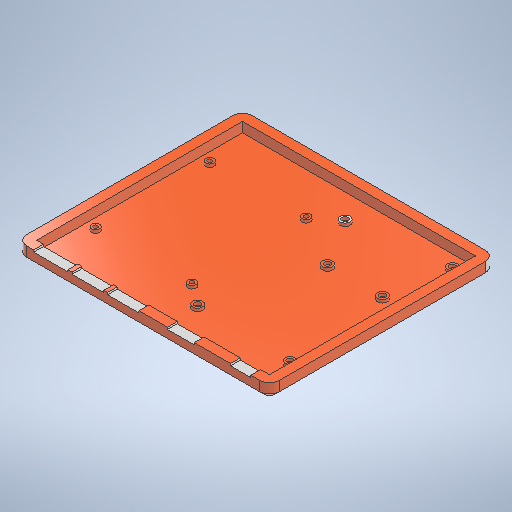
# Autodesk Inventor part: Electronic Base - Layered
Saved by Autodesk Inventor 2025.2 (Build 292293000, 293)
## iProperties
Created: 2025-02-05
Part Number: Electronic Base - Layered
Material: Generic
Document SubType Name: Modeling
Designer: caomi
Density: 1 g/cm^3
Appearance: Default
Author: caomi
Autodesk Inventor part; units mm, degrees
ref_plane "YZ Plane" through (0, 0, 0) normal (1, 0, 0) x (0, 1, 0)
ref_plane "XZ Plane" through (0, 0, 0) normal (0, 1, 0) x (-1, 0, 0)
ref_plane "XY Plane" through (0, 0, 0) normal (0, 0, 1) x (1, 0, 0)
sketch "Sketch1" plane through (0, 0, 0) normal (0, 1, 0) x (-1, 0, 0)
  line L0 (128.34, 114.6) -> (0, 114.6)
  line L1 (0, 114.6) -> (0, 0)
  line L2 (0, 0) -> (128.34, 0)
  line L3 (128.34, 0) -> (128.34, 114.6)
  line L4 (121.34, 23.6) -> (65.34, 23.6) construction
  line L5 (65.34, 23.6) -> (65.34, 108.6) construction
  line L6 (65.34, 108.6) -> (121.34, 108.6) construction
  line L7 (121.34, 108.6) -> (121.34, 23.6) construction
  circle A0 centre (117.84, 27.1) radius 1.1
  circle A1 centre (117.84, 85.1) radius 1.1
  circle A2 centre (68.84, 27.1) radius 1.1
  circle A3 centre (68.84, 85.1) radius 1.1
  line L8 (0, 0) -> (-136.9444, 0) construction
  line L9 (0, 0) -> (0, -49.9102) construction
  circle A4 centre (117.84, 27.1) radius 2.1
  circle A5 centre (117.84, 85.1) radius 2.1
  circle A6 centre (68.84, 27.1) radius 2.1
  circle A7 centre (68.84, 85.1) radius 2.1
  line L10 (123.34, 5) -> (5, 5)
  line L11 (5, 5) -> (5, 109.6)
  line L12 (5, 109.6) -> (123.34, 109.6)
  line L13 (123.34, 109.6) -> (123.34, 5)
  line L14 (60.34, 7) -> (7, 7) construction
  line L15 (7, 7) -> (7, 108.6) construction
  line L16 (7, 108.6) -> (60.34, 108.6) construction
  line L17 (60.34, 108.6) -> (60.34, 7) construction
  circle A8 centre (57.8, 18.43) radius 2.55
  circle A9 centre (57.8, 18.43) radius 1.55
  circle A10 centre (42.56, 42.56) radius 2.55
  circle A11 centre (42.56, 42.56) radius 1.55
  circle A12 centre (57.8, 93.36) radius 1.55
  circle A13 centre (14.62, 42.56) radius 2.55
  circle A14 centre (57.8, 93.36) radius 2.55
  circle A15 centre (14.62, 42.56) radius 1.55
  circle A16 centre (9.54, 12.08) radius 2.55
  circle A17 centre (9.54, 12.08) radius 1.55
  circle A18 centre (9.54, 94.63) radius 2.55
  circle A19 centre (9.54, 94.63) radius 1.55
  point P0 (121.34, 66.1)
  point P1 (7, 57.8)
  point P2 (1.5544, 63)
  point P3 (2.0056, 63)
  point P4 (82.8344, 63)
  point P5 (83.2856, 63)
  point P6 (33.67, 108.6)
  dimension "d10" = 2.2
  dimension "d48" = 101.6
  dimension "d49" = 53.34
  dimension "d59" = 5
  dimension "d62" = 3.1
  dimension "d63" = 1
  dimension "d73" = 5
  dimension "d79" = 5
  dimension "d81" = 2
  dimension "d82" = 2.54
  dimension "d83" = 15.24
  dimension "d84" = 90.17
  dimension "d85" = 96.52
  dimension "d86" = 50.8
  dimension "d87" = 66.04
  dimension "d88" = 17.78
  dimension "d89" = 45.72
  dimension "d90" = 13.97
  dimension "d91" = 85
  dimension "d92" = 58
  dimension "d95" = 1
  dimension "d96" = 3.5
  dimension "d97" = 3.5
  dimension "d98" = 3.5
  dimension "d99" = 56
  dimension "d100" = 2
  dimension "d101" = 2
  dimension "d102" = 5
  dimension "d103" = 5
  dimension "d120" = 1
  constraints: 36 end point, 20 centre point, 16 equal radius, 8 parallel, 6 coincident, 5 horizontal, 4 perpendicular, 4 vertical alignment, 3 horizontal alignment, 3 midpoint, 1 collinear, 1 vertical
  measures "d10" diameter of A0
  measures "d48" distance of L16.end L14.start
  measures "d49" distance of L15.end L16.end
  measures "d59" distance between parallel lines of L13 L3
  measures "d62" diameter of A9
  measures "d63" radial gap between concentric circles of A8 A9
  measures "d73" distance between parallel lines of L0 L12
  measures "d79" distance between parallel lines of L2 L10
  measures "d81" distance between parallel lines of L10 L14
  measures "d82" distance from line of L17 A12.centre
  measures "d83" distance from line of L16 A12.centre
  measures "d84" distance from line of L16 A9.centre
  measures "d85" distance from line of L16 A16.centre
  measures "d86" distance from line of L17 A17.centre
  measures "d87" distance from line of L16 A10.centre
  measures "d88" distance from line of L17 A10.centre
  measures "d89" distance from line of L17 A15.centre
  measures "d90" distance from line of L16 A18.centre
  measures "d91" distance of L4.end L5.end
  measures "d92" distance of A3.centre A2.centre
  measures "d95" radial gap between concentric circles of A4 A0
  measures "d96" distance from line of L4 A2.centre
  measures "d97" distance from line of L7 A0.centre
  measures "d98" distance from line of L5 A2.centre
  measures "d99" distance between parallel lines of L7 L5
  measures "d100" distance between parallel lines of L11 L15
  measures "d101" distance between parallel lines of L13 L7
  measures "d102" distance between parallel lines of L1 L11
  measures "d103" distance between parallel lines of L17 L5
  measures "d120" distance from line of L12 point (33.67, 108.6)
extrude "Extrusion1" add sketch "Sketch1" against normal blind 2 contours L3 L2 L1 L0 | A0 | A1 | A2 | A3 | A4 | A5 | A6 | A7 | L10 L11 L12 L13 | A8 | A9 | A10 | A11 | A12 | A13 | A14 | A15 | A16 | A17 | A18 | A19
extrude "Extrusion2" add sketch "Sketch1" along normal blind 5 contours L3 L2 L1 L0
extrude "Extrusion3" add sketch "Sketch1" along normal blind 1.5 contours A4 | A5 | A6 | A7 | A8 | A10 | A13 | A14 | A16 | A18
fillet "Fillet1" radius 5 4 edges at (-128.34, 1.5, 0) (0, 1.5, 114.6) (-128.34, 1.5, 114.6) (0, 1.5, 0)
chamfer "Chamfer1" distance 2 angle 45 7 edges at (-64.17, -2, 114.6) (-126.8755, -2, 113.1355) (-128.34, -2, 57.3) (-126.8755, -2, 1.4645) (-64.17, -2, 0) (0, -2, 57.3) (-1.4645, -2, 113.1355)
sketch "Sketch2" plane through (0, 5, 0) normal (0, 1, 0) x (1, 0, 0)
  line L0 (-123.34, -114.6) -> (-5, -114.6) projected
  line L1 (-5, -109.6) -> (-123.34, -109.6) projected
  line L2 (-119.84, -109.6) -> (-102.44, -109.6)
  line L3 (-102.44, -109.6) -> (-102.44, -114.6)
  line L4 (-102.44, -114.6) -> (-119.84, -114.6)
  line L5 (-119.84, -114.6) -> (-119.84, -109.6)
  line L6 (-100.34, -109.6) -> (-84.24, -109.6)
  line L7 (-84.24, -109.6) -> (-84.24, -114.6)
  line L8 (-84.24, -114.6) -> (-100.34, -114.6)
  line L9 (-100.34, -114.6) -> (-100.34, -109.6)
  line L10 (-82.34, -109.6) -> (-66.34, -109.6)
  line L11 (-66.34, -109.6) -> (-66.34, -114.6)
  line L12 (-66.34, -114.6) -> (-82.34, -114.6)
  line L13 (-82.34, -114.6) -> (-82.34, -109.6)
  line L14 (-51.84, -109.6) -> (-38.2, -109.6)
  line L15 (-38.2, -109.6) -> (-38.2, -114.6)
  line L16 (-38.2, -114.6) -> (-51.84, -114.6)
  line L17 (-51.84, -114.6) -> (-51.84, -109.6)
  line L18 (-121.34, -108.6) -> (-121.34, -23.6) construction
  line L19 (-60.34, -108.6) -> (-60.34, -7) construction
  line L20 (-19.84, -109.6) -> (-9.51, -109.6)
  line L21 (-9.51, -109.6) -> (-9.51, -114.6)
  line L22 (-9.51, -114.6) -> (-19.84, -114.6)
  line L23 (-19.84, -114.6) -> (-19.84, -109.6)
  point P0 (0, 0)
  point P1 (-9.51, -112.1)
  point P2 (-19.84, -114.6)
  point P3 (-51.84, -114.6)
  dimension "d104" = 17.4
  dimension "d107" = 16.1
  dimension "d109" = 16
  dimension "d113" = 13.64
  dimension "d114" = 1.5
  dimension "d115" = 21
  dimension "d116" = 39
  dimension "d117" = 8.5
  dimension "d118" = 40.5
  dimension "d119" = 10.33
  constraints: 40 end point, 10 parallel, 10 point on line, 5 horizontal, 5 perpendicular, 1 midpoint
  measures "d104" distance of L3.end L4.end
  measures "d107" distance of L7.end L8.end
  measures "d109" distance between parallel lines of L11 L13
  measures "d113" distance between parallel lines of L15 L17
  measures "d114" distance between parallel lines of L18 L5
  measures "d115" distance between parallel lines of L18 L9
  measures "d116" distance between parallel lines of L18 L13
  measures "d117" distance between parallel lines of L19 L17
  measures "d118" distance between parallel lines of L19 L23
  measures "d119" distance from line of point (-9.51, -112.1) L23
extrude "Extrusion4" cut sketch "Sketch2" against normal blind 1 contours L5 L1 L3 L0 | L9 L1 L7 L0 | L13 L1 L11 L0 | L17 L1 L15 L0 | L23 L1 L21 L0
equation "\"board_border\" = 2"
equation "\"base_wall\" = 5"
body "Solid1"
